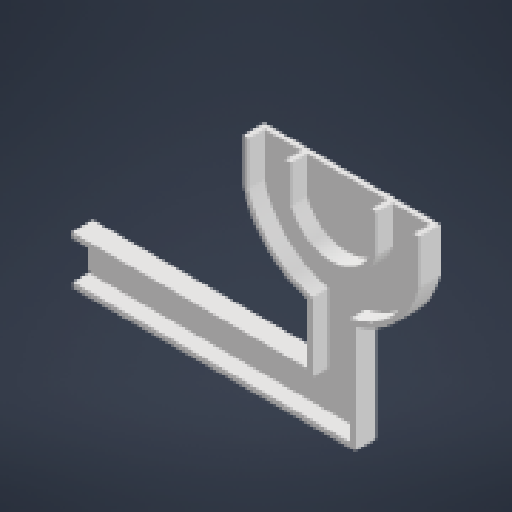
# Autodesk Inventor part: storrageout
Saved by Autodesk Inventor 2026.2 (Build 302298000, 298)
## iProperties
Created: 2026-04-16
Part Number: storrageout
Material: Generic
Document SubType Name: Modeling
Designer: danda
Density: 1 g/cm^3
Appearance: Default
Author: danda
Autodesk Inventor part; units mm, degrees
ref_plane "YZ Plane" through (0, 0, 0) normal (1, 0, 0) x (0, 1, 0)
ref_plane "XZ Plane" through (0, 0, 0) normal (0, 1, 0) x (-1, 0, 0)
ref_plane "XY Plane" through (0, 0, 0) normal (0, 0, 1) x (1, 0, 0)
sketch "Sketch1" plane through (0, 0, 0) normal (0, 0, 1) x (1, 0, 0)
  arc A0 (-37.5, -13.9194) -> (37.5, -13.9194) centre (0, 0) ccw
  line L0 (-37.5, -13.9194) -> (-37.5, 21.0806)
  line L1 (37.5, -13.9194) -> (37.5, 21.0806)
  arc A1 (-42.5, -14.7902) -> (42.5, -14.7902) centre (0, 0) ccw
  line L2 (-42.5, -14.7902) -> (-42.5, 21.0806)
  line L3 (42.5, -14.7902) -> (42.5, 21.0806)
  line L4 (77.5, 21.0806) -> (77.5, -19.8431)
  line L5 (-77.5, -19.8431) -> (-77.5, 21.0806)
  line L6 (82.5, 21.0806) -> (82.5, -20.4634)
  line L7 (-82.5, -20.4634) -> (-82.5, 21.0806)
  line L8 (17.5, -113.0625) -> (17.5, -78.0625)
  line L9 (-17.5, -113.0625) -> (-17.5, -78.0625)
  line L10 (22.5, -81.968) -> (22.5, -108.0625)
  line L11 (-22.5, -108.0625) -> (-22.5, -81.968)
  line L12 (22.5, -108.0625) -> (17.5, -108.0625)
  arc A2 (-77.5, -19.8431) -> (-17.5, -78.0625) centre (0, 0) ccw
  arc A3 (17.5, -78.0625) -> (77.5, -19.8431) centre (0, 0) ccw
  arc A4 (-82.5, -20.4634) -> (-22.5, -81.968) centre (0, 0) ccw
  arc A5 (22.5, -81.968) -> (82.5, -20.4634) centre (0, 0) ccw
  line L13 (-17.5, -113.0625) -> (-17.5, -108.0625)
  line L14 (17.5, -113.0625) -> (17.5, -108.0625)
  line L15 (-82.5, 21.0806) -> (-77.5, 21.0806)
  line L16 (-42.5, 21.0806) -> (-37.5, 21.0806)
  line L17 (37.5, 21.0806) -> (42.5, 21.0806)
  line L18 (77.5, 21.0806) -> (82.5, 21.0806)
  line L19 (-22.5, -13.9194) -> (-17.5, -13.9194)
  line L20 (17.5, -13.9194) -> (22.5, -13.9194)
  line L21 (-77.5, 21.0806) -> (82.5, 21.0806)
  line L22 (1.8649, -108.0625) -> (17.5, -108.0625)
  line L23 (22.5, -108.0625) -> (22.5, -143.0625)
  line L24 (17.5, -143.0625) -> (17.5, -108.0625)
  line L25 (-17.5, -108.0625) -> (-17.5, -113.0625)
  line L26 (22.5, -178.0625) -> (22.5, -178.0625)
  line L27 (-17.5, -183.0625) -> (-287.4597, -183.0625)
  line L28 (-17.5, -178.0625) -> (-287.099, -178.0625)
  line L29 (-287.4597, -138.0625) -> (-47.5, -138.0625)
  line L30 (-22.5, -113.0625) -> (-22.5, -108.0625)
  line L31 (-287.4597, -183.0625) -> (-287.4597, -138.0625)
  line L32 (-17.5, -78.0625) -> (17.5, -78.0625)
  line L33 (-243.2803, -138.0625) -> (-242.0268, -183.0625)
  arc A6 (-17.5, -178.0625) -> (17.5, -143.0625) centre (-17.5, -143.0625) ccw
  arc A7 (-17.5, -183.0625) -> (22.5, -143.0625) centre (-17.5, -143.0625) ccw
  arc A8 (-47.5, -143.0625) -> (-17.5, -113.0625) centre (-47.5, -113.0625) ccw
  arc A9 (-47.5, -138.0625) -> (-22.5, -113.0625) centre (-47.5, -113.0625) ccw
  line L34 (-47.5, -143.0625) -> (-287.4597, -143.0625)
  line L35 (-22.5, -113.0625) -> (-22.5, -108.0625)
  point P0 (-42.5, 21.0806)
  point P1 (77.5, 21.0806)
  point P2 (42.5, 21.0806)
  point P3 (17.5, -162.4274)
  point P4 (-287.5, -178.0625)
  point P5 (37.5, 21.0806)
  point P6 (-243.1411, -143.0625)
  point P7 (-242.1661, -178.0625)
  dimension "d0" = 75
  dimension "d1" = 40
  dimension "d2" = 35
  dimension "d3" = 35
  dimension "d4" = 5
  dimension "d5" = 5
  dimension "d6" = 5
  dimension "d9" = 35
  dimension "d10" = 20
  dimension "d11" = 5
  dimension "d12" = 0
  dimension "d13" = 0
  dimension "d14" = 5
  dimension "d21" = 35
  dimension "d22" = 310
  dimension "d23" = 305
  dimension "d24" = 5
  dimension "d31" = 100
  dimension "d32" = 85
  dimension "d33" = 80
  dimension "d34" = 78.0625
  dimension "d37" = 5
  constraints: 72 end point, 21 point on circle, 11 point on line, 10 centre point, 9 horizontal, 7 parallel, 6 vertical, 5 tangent, 1 coincident, 1 perpendicular
  measures "d0" distance of L0.start L1.start
  measures "d1" radius of A0
  measures "d2" distance of L0.start L0.end
  measures "d3" distance of L1.start L1.end
  measures "d4" radial gap between concentric circles of A0 A1
  measures "d5" distance between parallel lines of L0 L2
  measures "d6" distance between parallel lines of L1 L3
  measures "d9" distance of L9.start L8.start
  measures "d10" horizontal distance of L1.start L8.start
  measures "d11" distance between parallel lines of L7 L5
  measures "d12" distance of point (0, 0) A0.centre
  measures "d13" distance of point (0, 0) A0.centre
  measures "d14" distance between parallel lines of L8 L10
  measures "d21" distance of L23.end L26.end
  measures "d22" distance of L26.end L27.end
  measures "d23" distance of point (17.5, -162.427) L28.end
  measures "d24" distance between parallel lines of L27 L28
  measures "d31" distance between parallel lines of L28 L32
  measures "d32" radius of A4
  measures "d33" radius of A2
  measures "d34" distance from line of point (0, 0) L32
  measures "d37" radial gap between concentric circles of A8 A9
extrude "Extrusion1" add sketch "Sketch1" along normal blind 20 contours A0 L1 L17 L3 A1 L2 L16 L0 | L5 A2 L9 A8 L34 L33 L29 A9 L30 L11 A4 L7 L15 | L18 L6 A5 L10 L12 L8 A3 L4 | L12 L23 A7 L27 L33 L28 A6 L24 L8
extrude "Extrusion2" add sketch "Sketch1" along normal blind 5 contours L2 A1 L3 L21 L4 A3 L32 A2 L5 | L18 L6 A5 L10 L12 L8 A3 L4 | L32 L8 L24 A6 L28 L33 L34 A8 L9
extrude "Extrusion3" cut sketch "Sketch1" along normal through all both and the other way through all contours L34 L31 L29 L33 | L33 L27 L31 L34
equation "\"d3\" = d2"
body "Solid1"
